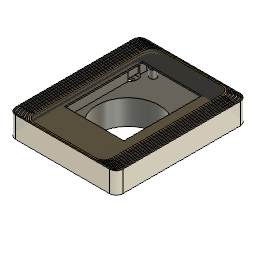
flush-mount-touch-display (Autodesk Fusion 360 design; units mm, degrees)
Autodesk Fusion 360 part; units mm, degrees
note: some values were not read from the file. Set by a fixed rule: which face or edge a step refers to.
(part 1 of 2)
sketch "Skizze2" plane through (0, 0, 0) normal (0, 0, 1) x (1, 0, 0)
  line L0 (0, 0) -> (50, 0)
  line L1 (50, 0) -> (50, 86)
  line L2 (50, 86) -> (0, 86)
  line L3 (0, 86) -> (0, 0)
  circle A0 centre (4.2, 5.1408) radius 1.25
  line L4 (25, 86) -> (25, 0) construction
  line L5 (0, 40) -> (50, 40) construction
  circle A1 centre (4.2, 5.1408) radius 2.5
  circle A2 centre (45.8, 5.1408) radius 1.25
  circle A3 centre (45.8, 5.1408) radius 2.5
  circle A4 centre (4.2, 82.6408) radius 1.25
  circle A5 centre (4.2, 82.6408) radius 2.5
  circle A6 centre (45.8, 82.6408) radius 2.5
  circle A7 centre (45.8, 82.6408) radius 1.25
  line L6 (43, 0) -> (7, 0)
  line L7 (7, 0) -> (7, 3.137)
  line L8 (7, 3.137) -> (43, 3.137)
  line L9 (43, 3.137) -> (43, 0)
  line L10 (43, 0) -> (7, 3.137) construction
  line L11 (7, 0) -> (43, 3.137) construction
  line L12 (50, 10) -> (0, 10) construction
  line L13 (0, 79.4) -> (50, 79.4) construction
  line L14 (0, 10) -> (0, 79.4) construction
  line L15 (0, 44.7) -> (50, 44.7) construction
  line L16 (2, -2) -> (48, -2)
  line L17 (52, 2) -> (52, 84)
  line L18 (48, 88) -> (2, 88)
  line L19 (-2, 84) -> (-2, 2)
  arc A8 (52, 84) -> (48, 88) centre (48, 84) ccw
  arc A9 (2, 88) -> (-2, 84) centre (2, 84) ccw
  arc A10 (-2, 2) -> (2, -2) centre (2, 2) ccw
  arc A11 (48, -2) -> (52, 2) centre (48, 2) ccw
  line L20 (-3.5, 84) -> (-3.5, 2)
  arc A12 (-3.5, 2) -> (2, -3.5) centre (2, 2) ccw
  line L21 (2, -3.5) -> (48, -3.5)
  arc A13 (48, -3.5) -> (53.5, 2) centre (48, 2) ccw
  line L22 (53.5, 2) -> (53.5, 84)
  arc A14 (53.5, 84) -> (48, 89.5) centre (48, 84) ccw
  line L23 (48, 89.5) -> (2, 89.5)
  arc A15 (2, 89.5) -> (-3.5, 84) centre (2, 84) ccw
  line L24 (7, 0) -> (7, -3.5)
  line L25 (43, 0) -> (43, -3.5)
  point P0 (25, 1.5685)
  dimension "d3" = 50
  dimension "d4" = 86
  dimension "d5" = 2.5
  dimension "d6" = 5
  dimension "d7" = 2.5
  dimension "d8" = 5
  dimension "d10" = 4
  dimension "d11" = 1.5
  dimension "d108" = 20.8
  dimension "d109" = 77.5
  dimension "d110" = 20.8
  constraint horizontal L0
  constraint vertical L1
  constraint horizontal L2
  constraint vertical L3
  constraint coincident L0.start L3.end
  constraint midpoint L2 L4.start
  constraint midpoint L0 L4.end
  constraint coincident L3 L5.start
  constraint coincident L1 L5.end
  constraint perpendicular L1 L5
  constraint concentric A0 A1
  constraint symmetric A0 L4 A2
  constraint symmetric L4 A1 A3
  constraint concentric A4 A5
  constraint symmetric L4 A4 A7
  constraint symmetric L4 A5 A6
  constraint horizontal L6
  constraint perpendicular L6 L7
  constraint parallel L6 L8
  constraint parallel L7 L9
  constraint coincident L10 P0
  constraint coincident L11 P0
  constraint coincident L0 L6.start
  constraint coincident L4 P0
  constraint coincident L1 L12.start
  constraint coincident L3 L12.end
  constraint perpendicular L3 L12
  constraint coincident L3 L13.start
  constraint coincident L1 L13.end
  constraint perpendicular L1 L13
  constraint midpoint L14 L15.start
  constraint coincident L1 L15.end
  constraint perpendicular L1 L15
  constraint tangent L17 A8
  constraint tangent L18 A8
  constraint tangent L18 A9
  constraint tangent L19 A9
  constraint equal A8 A9
  constraint tangent L16 A10
  constraint tangent L19 A10
  constraint equal A8 A10
  constraint tangent L16 A11
  constraint tangent L17 A11
  constraint equal A8 A11
  constraint coincident L21 L24.end
  constraint perpendicular L21 L24
  constraint coincident L21 L25.end
  constraint perpendicular L21 L25
  measures "d3" distance of L0.start L0.end
  measures "d4" distance of L0.start L2.end
  measures "d5" diameter of A0
  measures "d6" diameter of A1
  measures "d7" diameter of A4
  measures "d8" diameter of A5
  measures "d10" radius of A8
  measures "d108" distance of L4 A6.centre
  measures "d109" vertical distance of A2.centre A6.centre
  measures "d110" distance of L4 A2.centre
extrude "Extrusion1" add sketch "Skizze2" along normal blind 8.6 contours L16 L17 L18 L19 A8 A9 A10 A11 L20 A12 L21 A13 L22 A14 L23 A15 L24 L25 makes body 1
extrude "Extrusion2" add sketch "Skizze2" against normal blind 1.5 contours L0 L1 L2 L3 L7 L8 L9 | L0 L1 L2 L3 L16 L17 L18 L19 A8 A9 A10 A11 L24 L25 | L16 L17 L18 L19 A8 A9 A10 A11 L20 A12 L21 A13 L22 A14 L23 A15 L24 L25 | A0 | A1 | A2 | A3 | A4 | A5 | A6 | A7 bodies 1
extrude "Extrusion3" add sketch "Skizze2" along normal blind 4.2 contours A1 | A3 | A5 | A6 bodies 1
extrude "Extrusion4" add sketch "Skizze2" along normal blind 4.2 contours A0 | A2 | A4 | A7 bodies 1
sketch "Skizze3" plane through (0, 0, 0) normal (0, 0, 1) x (1, 0, 0)
  arc A0 (2, 89.5) -> (-3.5, 84) centre (2, 84) ccw
  line L0 (-3.5, 84) -> (-3.5, 2)
  arc A1 (-3.5, 2) -> (2, -3.5) centre (2, 2) ccw
  line L1 (2, -3.5) -> (48, -3.5)
  arc A2 (48, -3.5) -> (53.5, 2) centre (48, 2) ccw
  line L2 (53.5, 2) -> (53.5, 84)
  arc A3 (53.5, 84) -> (48, 89.5) centre (48, 84) ccw
  line L3 (48, 89.5) -> (2, 89.5)
  circle A4 centre (4.2, 82.6408) radius 2.5
  circle A5 centre (45.8, 82.6408) radius 2.5
  circle A6 centre (45.8, 5.1408) radius 2.5
  circle A7 centre (4.2, 5.1408) radius 2.5
  arc A8 (-3.55, 2) -> (2, -3.55) centre (2, 2) ccw
  line L4 (2, -3.55) -> (48, -3.55)
  arc A9 (48, -3.55) -> (53.55, 2) centre (48, 2) ccw
  line L5 (53.55, 2) -> (53.55, 84)
  arc A10 (53.55, 84) -> (48, 89.55) centre (48, 84) ccw
  line L6 (48, 89.55) -> (2, 89.55)
  arc A11 (2, 89.55) -> (-3.55, 84) centre (2, 84) ccw
  line L7 (-3.55, 84) -> (-3.55, 2)
  line L8 (48, 91.05) -> (2, 91.05)
  arc A12 (2, 91.05) -> (-5.05, 84) centre (2, 84) ccw
  line L9 (-5.05, 84) -> (-5.05, 2)
  arc A13 (-5.05, 2) -> (2, -5.05) centre (2, 2) ccw
  line L10 (2, -5.05) -> (48, -5.05)
  arc A14 (48, -5.05) -> (55.05, 2) centre (48, 2) ccw
  line L11 (55.05, 2) -> (55.05, 84)
  arc A15 (55.05, 84) -> (48, 91.05) centre (48, 84) ccw
  dimension "d26" = 0.05
  dimension "d27" = 1.55
extrude "Extrusion6" add sketch "Skizze3" against normal blind 1.8 separate body contours L8 A12 L9 A13 L10 A14 L11 A15 makes body 2
extrude "Extrusion7" add sketch "Skizze3" along normal blind 8.6 contours L8 A12 L9 A13 L10 A14 L11 A15 bodies 2
sketch "Skizze4" plane through (0, 0, 8.6) normal (0, 0, 1) x (-1, 0, 0)
  line L0 (3.55, -2) -> (3.55, -84)
  arc A0 (-2, -89.55) -> (3.55, -84) centre (-2, -84) ccw
  line L1 (-2, -89.55) -> (-48, -89.55)
  arc A1 (-53.55, -84) -> (-48, -89.55) centre (-48, -84) ccw
  line L2 (-53.55, -84) -> (-53.55, -2)
  arc A2 (-48, 3.55) -> (-53.55, -2) centre (-48, -2) ccw
  line L3 (-48, 3.55) -> (-2, 3.55)
  arc A3 (3.55, -2) -> (-2, 3.55) centre (-2, -2) ccw
  arc A4 (-55.05, -84) -> (-48, -91.05) centre (-48, -84) ccw
  line L4 (-48, -91.05) -> (-2, -91.05)
  arc A5 (-2, -91.05) -> (5.05, -84) centre (-2, -84) ccw
  line L5 (5.05, -84) -> (5.05, -2)
  arc A6 (5.05, -2) -> (-2, 5.05) centre (-2, -2) ccw
  line L6 (-2, 5.05) -> (-48, 5.05)
  arc A7 (-48, 5.05) -> (-55.05, -2) centre (-48, -2) ccw
  line L7 (-55.05, -2) -> (-55.05, -84)
  line L8 (5.05, -84) -> (5.05, -2)
  arc A8 (-2, -91.05) -> (5.05, -84) centre (-2, -84) ccw
  line L9 (-48, -91.05) -> (-2, -91.05)
  arc A9 (-55.05, -84) -> (-48, -91.05) centre (-48, -84) ccw
  line L10 (-55.05, -2) -> (-55.05, -84)
  arc A10 (-48, 5.05) -> (-55.05, -2) centre (-48, -2) ccw
  line L11 (-2, 5.05) -> (-48, 5.05)
  arc A11 (5.05, -2) -> (-2, 5.05) centre (-2, -2) ccw
  line L12 (0, -79.4) -> (-50, -79.4) construction
  line L13 (-50, -10) -> (0, -10) construction
  circle A12 centre (-4.2, -82.6408) radius 2.5
  circle A13 centre (-45.8, -82.6408) radius 2.5
  circle A14 centre (-45.8, -82.6408) radius 2.5
  circle A15 centre (-45.8, -5.1408) radius 2.5
  circle A16 centre (-45.8, -5.1408) radius 2.5
  circle A17 centre (-4.2, -5.1408) radius 2.5
  line L14 (0, -79.4) -> (0, -10) construction
  line L15 (-50, -79.4) -> (-50, -10) construction
  line L16 (0, -77.4) -> (-50, -77.4) construction
  line L17 (-50, -17.7) -> (0, -17.7) construction
  line L18 (-48, -79.4) -> (-48, -10) construction
  line L19 (-2, -79.4) -> (-2, -10) construction
  line L20 (-2, -77.4) -> (-48, -77.4)
  line L21 (-48, -77.4) -> (-48, -17.7)
  line L22 (-48, -17.7) -> (-2, -17.7)
  line L23 (-2, -17.7) -> (-2, -77.4)
  circle A18 centre (-45.8, -82.6408) radius 1.4
  circle A19 centre (-4.2, -82.6408) radius 1.4
  circle A20 centre (-45.8, -5.1408) radius 1.4
  circle A21 centre (-4.2, -5.1408) radius 1.4
  dimension "d32" = 2
  dimension "d33" = 7.7
  dimension "d34" = 2
  dimension "d35" = -2
  dimension "d44" = 2.8
  dimension "d45" = 2.8
  dimension "d46" = 2.8
  dimension "d47" = 2.8
  constraint coincident L12.start L14.start
  constraint coincident L13.end L14.end
  constraint coincident L12.end L15.start
  constraint coincident L13.start L15.end
  constraint horizontal L20
  constraint vertical L21
  constraint horizontal L22
  constraint vertical L23
  constraint coincident L18 L21.end
  constraint coincident L17 L21.end
  constraint coincident L19 L20.start
  constraint coincident L16 L20.start
  measures "d44" diameter of A18
  measures "d45" diameter of A19
  measures "d46" diameter of A20
  measures "d47" diameter of A21
extrude "Extrusion8" add sketch "Skizze4" along normal blind 1 contours L0 A0 L1 A1 L2 A2 L3 A3 | A4 L4 A5 L5 A6 L6 A7 L7 L8 A8 L9 A9 L10 A10 L11 A11 | A12 | A13 A14 | A15 A16 | A17 | A18 | A19 | A20 | A21 bodies 2
extrude "Extrusion9" add sketch "Skizze4" against normal blind 2.4 contours A12 | A13 A14 | A15 A16 | A17 | A18 | A19 | A20 | A21 bodies 2
sketch "Skizze5" plane through (0, 0, 9.6) normal (0, 0, 1) x (-1, 0, 0)
  line L0 (-48, -17.7) -> (-2, -17.7)
  line L1 (-2, -17.7) -> (-2, -77.4)
  line L2 (-2, -77.4) -> (-48, -77.4)
  line L3 (-48, -77.4) -> (-48, -17.7)
  arc A0 (5.05, -2) -> (-2, 5.05) centre (-2, -2) ccw
  line L4 (-2, 5.05) -> (-48, 5.05)
  arc A1 (-48, 5.05) -> (-55.05, -2) centre (-48, -2) ccw
  line L5 (-55.05, -2) -> (-55.05, -84)
  arc A2 (-55.05, -84) -> (-48, -91.05) centre (-48, -84) ccw
  line L6 (-48, -91.05) -> (-2, -91.05)
  arc A3 (-2, -91.05) -> (5.05, -84) centre (-2, -84) ccw
  line L7 (5.05, -84) -> (5.05, -2)
  line L8 (4.05, -84) -> (4.05, -2)
  arc A4 (4.05, -2) -> (-2, 4.05) centre (-2, -2) ccw
  line L9 (-2, 4.05) -> (-48, 4.05)
  arc A5 (-48, 4.05) -> (-54.05, -2) centre (-48, -2) ccw
  line L10 (-54.05, -2) -> (-54.05, -84)
  arc A6 (-54.05, -84) -> (-48, -90.05) centre (-48, -84) ccw
  line L11 (-48, -90.05) -> (-2, -90.05)
  arc A7 (-2, -90.05) -> (4.05, -84) centre (-2, -84) ccw
  line L12 (3.95, -84) -> (3.95, -2)
  arc A8 (3.95, -2) -> (-2, 3.95) centre (-2, -2) ccw
  line L13 (-2, 3.95) -> (-48, 3.95)
  arc A9 (-48, 3.95) -> (-53.95, -2) centre (-48, -2) ccw
  line L14 (-53.95, -2) -> (-53.95, -84)
  arc A10 (-53.95, -84) -> (-48, -89.95) centre (-48, -84) ccw
  line L15 (-48, -89.95) -> (-2, -89.95)
  arc A11 (-2, -89.95) -> (3.95, -84) centre (-2, -84) ccw
  dimension "d40" = -1
  dimension "d41" = -1.1
extrude "Extrusion10" cut sketch "Skizze5" against normal blind 0.1 contours L8 A4 L9 A5 L10 A6 L11 A7 bodies 2
sketch "Skizze6" plane through (0, 0, -1.5) normal (0, 0, -1) x (1, 0, 0)
  line L0 (7, -3.137) -> (7, 3.5)
  line L1 (7, 3.5) -> (2, 3.5)
  arc A0 (2, 3.5) -> (-3.5, -2) centre (2, -2) ccw
  line L2 (-3.5, -2) -> (-3.5, -84)
  arc A1 (-3.5, -84) -> (2, -89.5) centre (2, -84) ccw
  line L3 (2, -89.5) -> (48, -89.5)
  arc A2 (48, -89.5) -> (53.5, -84) centre (48, -84) ccw
  line L4 (53.5, -84) -> (53.5, -2)
  arc A3 (53.5, -2) -> (48, 3.5) centre (48, -2) ccw
  line L5 (48, 3.5) -> (43, 3.5)
  line L6 (43, 3.5) -> (43, -3.137)
  line L7 (43, -3.137) -> (7, -3.137)
  line L8 (2, 3.55) -> (48, 3.55)
  arc A4 (2, 3.55) -> (-3.55, -2) centre (2, -2) ccw
  arc A5 (53.55, -2) -> (48, 3.55) centre (48, -2) ccw
  line L9 (53.55, -2) -> (53.55, -84)
  arc A6 (48, -89.55) -> (53.55, -84) centre (48, -84) ccw
  line L10 (48, -89.55) -> (2, -89.55)
  arc A7 (-3.55, -84) -> (2, -89.55) centre (2, -84) ccw
  line L11 (-3.55, -84) -> (-3.55, -2)
  line L12 (25, 3.55) -> (25, -89.55) construction
  line L13 (-3.55, -43) -> (53.5, -43) construction
  line L14 (37, -79) -> (13, -79)
  line L15 (13, -79) -> (13, -7)
  line L16 (13, -7) -> (37, -7)
  line L17 (37, -7) -> (37, -79)
  line L18 (37, -79) -> (13, -7) construction
  line L19 (13, -79) -> (37, -7) construction
  circle A8 centre (28, -35) radius 3
  point P0 (25, -43)
  dimension "d49" = 24
  dimension "d121" = 6
  constraint midpoint L8 L12.start
  constraint midpoint L10 L12.end
  constraint midpoint L11 L13.start
  constraint midpoint L4 L13.end
  constraint horizontal L14
  constraint perpendicular L14 L15
  constraint parallel L14 L16
  constraint parallel L15 L17
  constraint coincident L18 P0
  constraint coincident L19 P0
  constraint midpoint L12 P0
  measures "d49" distance of L15.end L16.end
  measures "d121" diameter of A8
extrude "Extrusion11" add sketch "Skizze6" along normal blind 22 contours L14 L15 L16 L17 | A8 bodies 1
sketch "Skizze7" plane through (0, 79, 0) normal (0, 1, 0) x (-1, 0, 0)
  line L0 (-13, -1.5) -> (-37, -1.5)
  line L1 (-37, -1.5) -> (-37, -23.5)
  line L2 (-37, -23.5) -> (-13, -23.5)
  line L3 (-13, -23.5) -> (-13, -1.5)
  line L4 (-25, -23.5) -> (-25, -1.5) construction
  circle A0 centre (-25, -17) radius 12
  dimension "d52" = 24
  constraint midpoint L2 L4.start
  constraint midpoint L0 L4.end
  constraint coincident L4 A0.centre
  measures "d52" diameter of A0
extrude "Extrusion12" cut 1 faces at (21, 31, -23.5) along direction (0, 0, 1) blind 7 on bodies 1 bodies 1
fillet "Abrundung1" radius 12 1 edges at (25, 79, -16.5) on bodies 1
fillet "Abrundung2" radius 12 1 edges at (25, 7, -16.5) on bodies 1
extrude "Extrusion13" cut sketch "Skizze7" against normal blind 79 contours L2 A0 | L2 A0 bodies 1
sketch "Skizze16" plane through (0, 0, 0) normal (0, 0, 1) x (1, 0, 0)
  line L0 (37, 61) -> (13, 61)
  line L1 (13, 61) -> (13, 65)
  line L2 (13, 65) -> (37, 65)
  line L3 (37, 65) -> (37, 61)
  line L4 (37, 61) -> (13, 65) construction
  line L5 (13, 61) -> (37, 65) construction
  line L6 (37, 21) -> (13, 21)
  line L7 (13, 21) -> (13, 25)
  line L8 (13, 25) -> (37, 25)
  line L9 (37, 25) -> (37, 21)
  line L10 (37, 21) -> (13, 25) construction
  line L11 (13, 21) -> (37, 25) construction
  circle A0 centre (28, 35) radius 3
  line L12 (28, 38) -> (34, 38)
  line L13 (34, 38) -> (34, 32)
  line L14 (34, 32) -> (28, 32)
  line L15 (28, 32) -> (28, 38)
  line L16 (28, 38) -> (16, 38)
  line L17 (16, 38) -> (16, 32)
  line L18 (16, 32) -> (28, 32)
  line L19 (28, 32) -> (28, 38)
  point P0 (25, 63)
  point P1 (25, 23)
  constraint horizontal L0
  constraint perpendicular L0 L1
  constraint parallel L0 L2
  constraint parallel L1 L3
  constraint coincident L4 P0
  constraint coincident L5 P0
  constraint horizontal L6
  constraint perpendicular L6 L7
  constraint parallel L6 L8
  constraint parallel L7 L9
  constraint coincident L10 P1
  constraint coincident L11 P1
  constraint horizontal L12
  constraint vertical L13
  constraint horizontal L14
  constraint vertical L15
  constraint coincident A0 L12.start
  constraint horizontal L16
  constraint vertical L17
  constraint horizontal L18
  constraint vertical L19
extrude "Extrusion25" add 1 faces at (-3, 56.6667, 8.6) along direction (0, 0, 1) blind 0.9 on bodies 1 bodies 1
move_body "Verschieben1" bodies 2 to x (1, 0, 0) y (0, 1, 0) z (0, 0, 1) at (0, 0, 0.9)
extrude "Extrusion26" add 1 faces at (54.55, 29.3333, -0.9) along direction (0, 0, -1) blind 0.9 on bodies 2 bodies 2
extrude "Extrusion27" add sketch "Skizze2" along normal blind 8 contours A0 | A2 | A4 | A7 bodies 1
extrude "Extrusion28" add sketch "Skizze4" along normal blind 1 contours A12 | A13 A14 | A15 A16 | A17 bodies 2
extrude "Extrusion29" add sketch "Skizze4" against normal blind 2.8 contours A12 | A13 A14 | A15 A16 | A17 bodies 2
sketch "Skizze17" plane through (0, 0, 0) normal (0, 0, 1) x (1, 0, 0)
  line L0 (17, 32, -33) -> (33, 32, -33)
  line L1 (33, 32, -33) -> (33, 38, -33)
  line L2 (33, 38, -33) -> (17, 38, -33)
  line L3 (17, 38, -33) -> (17, 32, -33)
extrude "Extrusion34" cut 4 faces at (3.9935, 4.8544, 7.1) (3.9667, 82.2367, 7.1) (45.5667, 83.045, 7.1) (46.4103, 4.7622, 7.1) along direction (0, 0, 1) blind 1.5 on bodies 2 bodies 2
copy_body "Körper->Berechn1" bodies 1 removing the originals makes body 3 in component "Inner Body"
copy_body "Körper->Berechn2" bodies 2 removing the originals makes body 4 in component "Outer Body"
sketch "Skizze18" plane through (0, 0, 0) normal (0, 1, 0) x (1, 0, 0)
sketch "Skizze19" plane through (-5.05, 0, 0) normal (-1, 0, 0) x (0, -1, 0)
  line L0 (-84, 10.5) -> (-84, -1.8)
  line L1 (-84, -1.8) -> (-2, -1.8)
  line L2 (-2, -1.8) -> (-2, 10.5)
  line L3 (-2, 10.5) -> (-84, 10.5)
delete_face "Fläche löschen1" 1 faces at (37, 35, -6.5) on bodies 3 in component "Inner Body"
sketch "Skizze20" plane through (0, 0, 0) normal (0, 0, 1) x (-1, 0, 0)
  circle A0 centre (-4.2, -82.6408) radius 2.5
  circle A1 centre (-45.8, -82.6408) radius 2.5
  line L0 (-2, 2) -> (-7, 2)
  line L1 (-7, 2) -> (-7, -3.137)
  line L2 (-7, -3.137) -> (-43, -3.137)
  line L3 (-43, -3.137) -> (-43, 2)
  line L4 (-43, 2) -> (-48, 2)
  arc A2 (-48, 2) -> (-52, -2) centre (-48, -2) ccw
  line L5 (-52, -2) -> (-52, -84)
  arc A3 (-52, -84) -> (-48, -88) centre (-48, -84) ccw
  line L6 (-48, -88) -> (-2, -88)
  arc A4 (-2, -88) -> (2, -84) centre (-2, -84) ccw
  line L7 (2, -84) -> (2, -2)
  arc A5 (2, -2) -> (-2, 2) centre (-2, -2) ccw
  circle A6 centre (-4.2, -5.1408) radius 2.5
  circle A7 centre (-45.8, -5.1408) radius 2.5
  circle A8 centre (-25, -43.4454) radius 6
  line L8 (-4.2, -82.6408) -> (-12.2, -82.6408) construction
  line L9 (-12.2, -82.6408) -> (-12.2, -74.6408) construction
  circle A9 centre (-12.2, -74.6408) radius 2.1
  line L10 (-25, -88) -> (-25, -5.1408) construction
  line L11 (-4.2, -5.1408) -> (-12.2, -5.1408) construction
  line L12 (-12.2, -5.1408) -> (-12.2, -13.1408) construction
  circle A10 centre (-12.2, -13.1408) radius 2.1
  circle A11 centre (-37.8, -13.1408) radius 2.1
  circle A12 centre (-37.8, -74.6408) radius 2.1
  dimension "d152" = 12
  dimension "d155" = 8
  dimension "d156" = 8
  dimension "d157" = 4.2
  dimension "d158" = 8
  dimension "d159" = 8
  dimension "d160" = 4.2
  constraint coincident A0.centre L8.start
  constraint perpendicular L8 L9
  constraint coincident L9.end A9.centre
  constraint midpoint L6 L10.start
  constraint perpendicular L2 L10
  constraint coincident A6.centre L11.start
  constraint perpendicular L7 L11
  constraint perpendicular L11 L12
  constraint coincident L12.end A10.centre
  constraint symmetric A9 L10 A12
  constraint symmetric L10 A10 A11
  measures "d152" diameter of A8
  measures "d155" distance of A0.centre L8.end
  measures "d156" distance of L8.end L9.end
  measures "d157" diameter of A9
  measures "d158" distance of A6.centre L11.end
  measures "d159" distance of L11.end L12.end
  measures "d160" diameter of A10
extrude "Extrusion2'" cut sketch "Skizze20" against normal blind 5 contours A8 | A9 | A10 | A11 | A12 bodies 3 in component "Inner Body"
sketch "Skizze21" plane through (0, 0, 0) normal (0, 0, 1) x (-1, 0, 0)
  circle A0 centre (-25, -43.4454) radius 6
  circle A1 centre (-37.8, -74.6408) radius 2.1
  circle A2 centre (-37.8, -13.1408) radius 2.1
  circle A3 centre (-12.2, -74.6408) radius 2.1
  circle A4 centre (-12.2, -13.1408) radius 2.1
  circle A5 centre (-4.2, -82.6408) radius 2.5
  circle A6 centre (-45.8, -82.6408) radius 2.5
  line L0 (-2, 2) -> (-7, 2)
  line L1 (-7, 2) -> (-7, -3.137)
  line L2 (-7, -3.137) -> (-43, -3.137)
  line L3 (-43, -3.137) -> (-43, 2)
  line L4 (-43, 2) -> (-48, 2)
  arc A7 (-48, 2) -> (-52, -2) centre (-48, -2) ccw
  line L5 (-52, -2) -> (-52, -84)
  arc A8 (-52, -84) -> (-48, -88) centre (-48, -84) ccw
  line L6 (-48, -88) -> (-2, -88)
  arc A9 (-2, -88) -> (2, -84) centre (-2, -84) ccw
  line L7 (2, -84) -> (2, -2)
  arc A10 (2, -2) -> (-2, 2) centre (-2, -2) ccw
  circle A11 centre (-4.2, -5.1408) radius 2.5
  circle A12 centre (-45.8, -5.1408) radius 2.5
  line L8 (-25, -88) -> (-25, 3) construction
  line L9 (-52, -43) -> (2, -43) construction
  line L10 (5.45, -7.55) -> (-55.45, -7.55)
  line L11 (-60.45, -12.55) -> (-60.45, -73.45)
  line L12 (-55.45, -78.45) -> (5.45, -78.45)
  line L13 (10.45, -73.45) -> (10.45, -12.55)
  line L14 (10.45, -7.55) -> (-60.45, -78.45) construction
  line L15 (-60.45, -7.55) -> (10.45, -78.45) construction
  arc A13 (-60.45, -73.45) -> (-55.45, -78.45) centre (-55.45, -73.45) ccw
  arc A14 (5.45, -78.45) -> (10.45, -73.45) centre (5.45, -73.45) ccw
  arc A15 (10.45, -12.55) -> (5.45, -7.55) centre (5.45, -12.55) ccw
  arc A16 (-55.45, -7.55) -> (-60.45, -12.55) centre (-55.45, -12.55) ccw
  line L16 (3.55, -84) -> (3.55, -2)
  arc A17 (3.55, -2) -> (-2, 3.55) centre (-2, -2) ccw
  line L17 (-2, 3.55) -> (-48, 3.55)
  arc A18 (-48, 3.55) -> (-53.55, -2) centre (-48, -2) ccw
  line L18 (-53.55, -2) -> (-53.55, -84)
  arc A19 (-53.55, -84) -> (-48, -89.55) centre (-48, -84) ccw
  line L19 (-48, -89.55) -> (-2, -89.55)
  arc A20 (-2, -89.55) -> (3.55, -84) centre (-2, -84) ccw
  arc A21 (-55.05, -84) -> (-48, -91.05) centre (-48, -84) ccw
  line L20 (-55.05, -84) -> (-55.05, -2)
  arc A22 (-48, 5.05) -> (-55.05, -2) centre (-48, -2) ccw
  line L21 (-48, 5.05) -> (-2, 5.05)
  arc A23 (5.05, -2) -> (-2, 5.05) centre (-2, -2) ccw
  line L22 (5.05, -2) -> (5.05, -84)
  arc A24 (-2, -91.05) -> (5.05, -84) centre (-2, -84) ccw
  line L23 (-2, -91.05) -> (-48, -91.05)
  line L24 (-65.25, -83.25) -> (15.25, -83.25)
  line L25 (15.25, -83.25) -> (15.25, -2.75)
  line L26 (15.25, -2.75) -> (-65.25, -2.75)
  line L27 (-65.25, -2.75) -> (-65.25, -83.25)
  line L28 (-65.25, -83.25) -> (15.25, -2.75) construction
  line L29 (15.25, -83.25) -> (-65.25, -2.75) construction
  line L30 (-60.25, -92.0661) -> (10.25, -92.0661)
  line L31 (15.25, -87.0661) -> (15.25, 1.0661)
  line L32 (10.25, 6.0661) -> (-60.25, 6.0661)
  line L33 (-65.25, 1.0661) -> (-65.25, -87.0661)
  line L34 (-65.25, -92.0661) -> (15.25, 6.0661) construction
  line L35 (15.25, -92.0661) -> (-65.25, 6.0661) construction
  arc A25 (10.25, -92.0661) -> (15.25, -87.0661) centre (10.25, -87.0661) ccw
  arc A26 (-65.25, -87.0661) -> (-60.25, -92.0661) centre (-60.25, -87.0661) ccw
  arc A27 (-60.25, 6.0661) -> (-65.25, 1.0661) centre (-60.25, 1.0661) ccw
  arc A28 (15.25, 1.0661) -> (10.25, 6.0661) centre (10.25, 1.0661) ccw
  line L36 (-55.23, -84) -> (-55.23, -2)
  arc A29 (-48, 5.23) -> (-55.23, -2) centre (-48, -2) ccw
  line L37 (-48, 5.23) -> (-2, 5.23)
  arc A30 (5.23, -2) -> (-2, 5.23) centre (-2, -2) ccw
  line L38 (5.23, -2) -> (5.23, -84)
  arc A31 (-2, -91.23) -> (5.23, -84) centre (-2, -84) ccw
  line L39 (-2, -91.23) -> (-48, -91.23)
  arc A32 (-55.23, -84) -> (-48, -91.23) centre (-48, -84) ccw
  circle A33 centre (-25, -43) radius 26.75
  point P0 (-25, -43.8908)
  point P1 (-25, -43.8908)
  point P2 (-25, -43)
  point P3 (-25, -43)
  point P4 (-25, -43)
  dimension "d167" = 70.9
  dimension "d168" = 70.9
  dimension "d169" = 5
  dimension "d170" = 80.5
  dimension "d171" = 80.5
  dimension "d172" = 5
  dimension "d173" = 0.18
  dimension "d180" = 53.5
  constraint coincident P1 P0
  constraint midpoint L6 L8.start
  constraint perpendicular L2 L8
  constraint midpoint L5 L9.start
  constraint midpoint L7 L9.end
  constraint horizontal L10
  constraint perpendicular L10 L11
  constraint parallel L10 L12
  constraint parallel L11 L13
  constraint coincident L14 P4
  constraint coincident L15 P4
  constraint midpoint L9 P4
  constraint coincident L14.end L11
  constraint coincident L14.end L12
  constraint tangent L11 A13
  constraint tangent L12 A13
  constraint coincident L15.end L12
  constraint coincident L15.end L13
  constraint tangent L12 A14
  constraint tangent L13 A14
  constraint equal A13 A14
  constraint coincident L14.start L10
  constraint coincident L14.start L13
  constraint tangent L10 A15
  constraint tangent L13 A15
  constraint equal A13 A15
  constraint coincident L15.start L10
  constraint coincident L15.start L11
  constraint tangent L10 A16
  constraint tangent L11 A16
  constraint equal A13 A16
  constraint horizontal L24
  constraint perpendicular L24 L25
  constraint parallel L24 L26
  constraint parallel L25 L27
  constraint coincident L28 P4
  constraint coincident L29 P4
  constraint coincident P4 P3
  constraint horizontal L30
  constraint perpendicular L30 L31
  constraint parallel L30 L32
  constraint parallel L31 L33
  constraint coincident L34 P4
  constraint coincident L35 P4
  constraint coincident L35.start L30
  constraint coincident L35.start L31
  constraint tangent L30 A25
  constraint tangent L31 A25
  constraint coincident L34.start L33
  constraint coincident L34.start L30
  constraint tangent L33 A26
  constraint tangent L30 A26
  constraint equal A25 A26
  constraint coincident L35.end L33
  constraint coincident L35.end L32
  constraint tangent L33 A27
  constraint tangent L32 A27
  constraint equal A25 A27
  constraint coincident L34.end L32
  constraint coincident L34.end L31
  constraint tangent L32 A28
  constraint tangent L31 A28
  constraint equal A25 A28
  measures "d167" distance of L14.end L15.end
  measures "d168" distance of L15.start L14.end
  measures "d169" radius of A13
  measures "d170" distance of L25.end L26.end
  measures "d171" distance of L24.end L25.end
  measures "d172" radius of A25
  measures "d180" diameter of A33
extrude "Extrusion37" add sketch "Skizze21" against normal blind 2.5 separate body contours A0 | A1 | A2 | A3 | A4 | A5 L24 | A5 A6 L5 L7 L12 L24 | A5 L24 | A5 A6 L5 A8 L6 A9 L7 L24 | A6 L24 | A6 L24 | L5 A8 L6 A9 L7 L16 L18 A19 L19 A20 L24 | L7 L12 L16 L24 | L5 L7 A11 A12 L10 L12 | L7 L10 L12 L16 | L16 L18 A19 L19 A20 A21 L20 L22 A24 L23 L24 | L12 L16 L22 L24 | L5 L12 L18 L24 | L7 A11 L10 L26 | L7 L10 L16 L26 | L5 L10 L12 L18 | L10 L12 L16 L22 | A21 L20 L22 A24 L23 L24 L36 L38 A31 L39 A32 | L12 L22 L24 L38 | L12 L18 L20 L24 | L0 L1 L7 A10 A11 L26 | L0 L1 L3 L4 A7 L5 L7 A10 L16 A17 L17 A18 L18 L26 | L10 L16 L22 L26 | A11 L10 L26 | A11 L10 | L5 L10 L18 L26 | L5 A12 L10 L26 | L10 L12 L18 L20 | L10 L12 L22 L38 | L10 L12 L13 A14 A15 L24 L25 L26 L31 L38 | L24 L30 L31 L33 A25 A26 L36 L38 A31 L39 A32 | L12 L20 L24 L36 | L16 A17 L17 A18 L18 L20 A22 L21 A23 L22 L26 | A11 L26 | L10 L22 L26 L38 | L1 L2 L3 A11 A12 L10 L26 | L3 L4 A7 L5 A12 L26 | A12 L10 | A12 L10 L26 | L10 L18 L20 L26 | L10 L12 L20 L36 | L10 L12 L13 A14 A15 L38 | L10 L11 L12 A13 A16 L24 L26 L27 L33 L36 | L20 A22 L21 A23 L22 L26 L36 A29 L37 A30 L38 | A12 L26 | L10 L20 L26 L36 | L10 L11 L12 A13 A16 L36 | L26 L31 L32 L33 A27 A28 L36 A29 L37 A30 L38 | L1 L2 L3 L26 | A33 makes body 5
extrude "Extrusion38" cut sketch "Skizze21" against normal blind 1.8 contours L16 L18 A19 L19 A20 A21 L20 L22 A24 L23 L24 | L12 L16 L22 L24 | L10 L12 L16 L22 | L12 L18 L20 L24 | L10 L16 L22 L26 | L10 L12 L18 L20 | L16 A17 L17 A18 L18 L20 A22 L21 A23 L22 L26 | L10 L18 L20 L26 bodies 5
extrude "Extrusion39" cut sketch "Skizze21" against normal blind 18 contours A0 | A33 bodies 5
extrude "Extrusion3'" cut sketch "Skizze21" against normal blind 18 contours A0 | A33 bodies 3 in component "Inner Body"
sketch "Skizze22" plane through (0, 0, -2.5) normal (0, 0, -1) x (1, 0, 0)
  circle A0 centre (25, -43) radius 26.75
  line L0 (60.25, 6.0661) -> (-10.25, 6.0661)
  arc A1 (-10.25, 6.0661) -> (-15.25, 1.0661) centre (-10.25, 1.0661) ccw
  line L1 (-15.25, 1.0661) -> (-15.25, -87.0661)
  arc A2 (-15.25, -87.0661) -> (-10.25, -92.0661) centre (-10.25, -87.0661) ccw
  line L2 (-10.25, -92.0661) -> (60.25, -92.0661)
  arc A3 (60.25, -92.0661) -> (65.25, -87.0661) centre (60.25, -87.0661) ccw
  line L3 (65.25, -87.0661) -> (65.25, 1.0661)
  arc A4 (65.25, 1.0661) -> (60.25, 6.0661) centre (60.25, 1.0661) ccw
  line L4 (60.45, -12.55) -> (60.45, -73.45)
  arc A5 (55.45, -78.45) -> (60.45, -73.45) centre (55.45, -73.45) ccw
  line L5 (55.45, -78.45) -> (-5.45, -78.45)
  arc A6 (-10.45, -73.45) -> (-5.45, -78.45) centre (-5.45, -73.45) ccw
  line L6 (-10.45, -73.45) -> (-10.45, -12.55)
  arc A7 (-5.45, -7.55) -> (-10.45, -12.55) centre (-5.45, -12.55) ccw
  line L7 (-5.45, -7.55) -> (55.45, -7.55)
  arc A8 (60.45, -12.55) -> (55.45, -7.55) centre (55.45, -12.55) ccw
  circle A9 centre (25, -43) radius 26.75
  ellipse E0 centre (55.45, -73.45) end of major axis (53, -76) minor radius 1.9
  line L8 (57.9, -70.9) -> (53, -76) construction
  line L9 (54.0799, -72.1336) -> (56.8201, -74.7664) construction
  ellipse E1 centre (55.45, -12.55) end of major axis (58, -15) minor radius 1.9
  ellipse E2 centre (-5.45, -12.55) end of major axis (-3, -10) minor radius 1.9
  ellipse E3 centre (-5.45, -73.45) end of major axis (-8, -71) minor radius 1.9
  dimension "d185" = 3.8
  dimension "d187" = 360
  constraint coincident E0 L8.start
  constraint coincident E0 L8.end
  constraint coincident E0 L9.start
  constraint coincident E0 L9.end
  constraint concentric A5 E0
extrude "Extrusion40" add sketch "Skizze22" along normal blind 3 contours L0 A1 L1 A2 L2 A3 L3 A4 | L4 A5 L5 A6 L6 A7 L7 A8 bodies 5
sketch "Skizze23" plane through (0, 0, 0) normal (0, 0, 1) x (-1, 0, 0)
  arc A0 (-60.25, 6.0661) -> (-65.25, 1.0661) centre (-60.25, 1.0661) ccw
  line L0 (-65.25, 1.0661) -> (-65.25, -87.0661)
  arc A1 (-65.25, -87.0661) -> (-60.25, -92.0661) centre (-60.25, -87.0661) ccw
  line L1 (-60.25, -92.0661) -> (10.25, -92.0661)
  arc A2 (10.25, -92.0661) -> (15.25, -87.0661) centre (10.25, -87.0661) ccw
  line L2 (15.25, -87.0661) -> (15.25, 1.0661)
  arc A3 (15.25, 1.0661) -> (10.25, 6.0661) centre (10.25, 1.0661) ccw
  line L3 (10.25, 6.0661) -> (-60.25, 6.0661)
  line L4 (-48, 5.05) -> (-2, 5.05)
  arc A4 (5.05, -2) -> (-2, 5.05) centre (-2, -2) ccw
  line L5 (5.05, -2) -> (5.05, -84)
  arc A5 (-2, -91.05) -> (5.05, -84) centre (-2, -84) ccw
  line L6 (-2, -91.05) -> (-48, -91.05)
  arc A6 (-55.05, -84) -> (-48, -91.05) centre (-48, -84) ccw
  line L7 (-55.05, -84) -> (-55.05, -2)
  arc A7 (-48, 5.05) -> (-55.05, -2) centre (-48, -2) ccw
  ellipse E0 centre (5.45, -12.55) end of major axis (3, -10) minor radius 1.9
  ellipse E1 centre (-55.45, -12.55) end of major axis (-58, -15) minor radius 1.9
  ellipse E2 centre (-55.45, -73.45) end of major axis (-53, -76) minor radius 1.9
  ellipse E3 centre (5.45, -73.45) end of major axis (8, -71) minor radius 1.9
  ellipse E4 centre (5.45, -73.45) end of major axis (10.1633, -68.9215) minor radius 4.9
  ellipse E5 centre (-55.45, -73.45) end of major axis (-50.9215, -78.1633) minor radius 4.9
  ellipse E6 centre (-55.45, -12.55) end of major axis (-60.1633, -17.0785) minor radius 4.9
  ellipse E7 centre (5.45, -12.55) end of major axis (0.9215, -7.8367) minor radius 4.9
extrude "Extrusion41" cut sketch "Skizze23" against normal blind 4 contours L7 E1 E6 | L7 E1 E6 | L5 E0 E7 | L5 E0 E7 | L7 E1 | L7 E1 | L5 E0 | L5 E0 | L7 E2 E5 | L7 E2 E5 | L5 E3 E4 | L5 E3 E4 | L7 E2 | L7 E2 | L5 E3 | L5 E3 bodies 5
extrude "Extrusion4'" cut sketch "Skizze23" along normal blind 11 and the other way blind 4 contours L7 E1 E6 | L7 E1 E6 | L5 E0 E7 | L5 E0 E7 | L7 E1 | L7 E1 | L5 E0 | L5 E0 | L7 E2 E5 | L7 E2 E5 | L5 E3 E4 | L5 E3 E4 | L7 E2 | L7 E2 | L5 E3 | L5 E3 bodies 3 in component "Inner Body"
sketch "Skizze24" plane through (0, 0, -5.5) normal (0, 0, -1) x (1, 0, 0)
  ellipse E0 centre (-5.45, -12.55) end of major axis (-3, -10) minor radius 1.9
  ellipse E1 centre (-5.45, -73.45) end of major axis (-8, -71) minor radius 1.9
  circle A0 centre (25, -43) radius 26.75
  ellipse E2 centre (55.45, -12.55) end of major axis (58, -15) minor radius 1.9
  ellipse E3 centre (55.45, -73.45) end of major axis (53, -76) minor radius 1.9
  arc A1 (65.25, 1.0661) -> (60.25, 6.0661) centre (60.25, 1.0661) ccw
  line L0 (60.25, 6.0661) -> (-10.25, 6.0661)
  arc A2 (-10.25, 6.0661) -> (-15.25, 1.0661) centre (-10.25, 1.0661) ccw
  line L1 (-15.25, 1.0661) -> (-15.25, -87.0661)
  arc A3 (-15.25, -87.0661) -> (-10.25, -92.0661) centre (-10.25, -87.0661) ccw
  line L2 (-10.25, -92.0661) -> (60.25, -92.0661)
  arc A4 (60.25, -92.0661) -> (65.25, -87.0661) centre (60.25, -87.0661) ccw
  line L3 (65.25, -87.0661) -> (65.25, 1.0661)
  circle A5 centre (25, -43) radius 26.75
  circle A6 centre (25, -43) radius 28.75
  dimension "d196" = 2
extrude "Extrusion42" add sketch "Skizze24" along normal blind 30 contours A6 bodies 5
sketch "Skizze25" plane through (0, 0, -35.5) normal (0, 0, -1) x (1, 0, 0)
  circle A0 centre (25, -43) radius 26.75
  circle A1 centre (25, -43) radius 28.75
  circle A2 centre (25, -43) radius 28.75
  circle A3 centre (25, -43) radius 15
  dimension "d201" = 30
  constraint concentric A2 A3
  measures "d201" diameter of A3
extrude "Extrusion43" add sketch "Skizze25" against normal blind 2 contours A0 | A1 A2 | A3 bodies 5
extrude "Extrusion44" cut sketch "Skizze25" against normal blind 11 contours A3 bodies 5
extrude "Extrusion45" cut 1 faces at (59.4089, 3.0609, 0) along direction (0, 0, -1) blind 1.9 on bodies 5 bodies 5
extrude "Extrusion46" add 1 faces at (59.4089, 3.0609, -1.9) along direction (0, 0, 1) blind 0.1 on bodies 5 bodies 5
sketch "Skizze26" plane through (0, 0, -1.8) normal (0, 0, 1) x (-1, 0, 0)
  arc A0 (15.25, 1.0661) -> (10.25, 6.0661) centre (10.25, 1.0661) ccw
  line L0 (10.25, 6.0661) -> (-60.25, 6.0661)
  arc A1 (-60.25, 6.0661) -> (-65.25, 1.0661) centre (-60.25, 1.0661) ccw
  line L1 (-65.25, 1.0661) -> (-65.25, -87.0661)
  arc A2 (-65.25, -87.0661) -> (-60.25, -92.0661) centre (-60.25, -87.0661) ccw
  line L2 (-60.25, -92.0661) -> (10.25, -92.0661)
  arc A3 (10.25, -92.0661) -> (15.25, -87.0661) centre (10.25, -87.0661) ccw
  line L3 (15.25, -87.0661) -> (15.25, 1.0661)
  ellipse E0 centre (-55.45, -12.55) end of major axis (-60.1633, -17.0785) minor radius 4.9 (-53.55, -6.8131) -> (-53.55, -17.234) ccw
  line L4 (-53.55, -6.8131) -> (-53.55, -2)
  arc A4 (-48, 3.55) -> (-53.55, -2) centre (-48, -2) ccw
  line L5 (-48, 3.55) -> (-2, 3.55)
  arc A5 (3.55, -2) -> (-2, 3.55) centre (-2, -2) ccw
  line L6 (3.55, -2) -> (3.55, -6.7496)
  ellipse E1 centre (5.45, -12.55) end of major axis (0.9215, -7.8367) minor radius 4.9 (3.55, -17.2737) -> (3.55, -6.7496) ccw
  line L7 (3.55, -17.2737) -> (3.55, -68.766)
  ellipse E2 centre (5.45, -73.45) end of major axis (10.1633, -68.9215) minor radius 4.9 (3.55, -79.1869) -> (3.55, -68.766) ccw
  line L8 (3.55, -79.1869) -> (3.55, -84)
  arc A6 (-2, -89.55) -> (3.55, -84) centre (-2, -84) ccw
  line L9 (-2, -89.55) -> (-48, -89.55)
  arc A7 (-53.55, -84) -> (-48, -89.55) centre (-48, -84) ccw
  line L10 (-53.55, -84) -> (-53.55, -79.2504)
  ellipse E3 centre (-55.45, -73.45) end of major axis (-50.9215, -78.1633) minor radius 4.9 (-53.55, -68.7263) -> (-53.55, -79.2504) ccw
  line L11 (-53.55, -68.7263) -> (-53.55, -17.234)
sketch "Skizze27" plane through (0, 0, 10.5) normal (0, 0, 1) x (-1, 0, 0)
  line L0 (-48, -89.95) -> (-2, -89.95)
  arc A0 (-2, -89.95) -> (3.95, -84) centre (-2, -84) ccw
  line L1 (3.95, -84) -> (3.95, -2)
  arc A1 (3.95, -2) -> (-2, 3.95) centre (-2, -2) ccw
  line L2 (-2, 3.95) -> (-48, 3.95)
  arc A2 (-48, 3.95) -> (-53.95, -2) centre (-48, -2) ccw
  line L3 (-53.95, -2) -> (-53.95, -84)
  arc A3 (-53.95, -84) -> (-48, -89.95) centre (-48, -84) ccw
  line L4 (-48, -17.7) -> (-2, -17.7)
  line L5 (-2, -17.7) -> (-2, -77.4)
  line L6 (-2, -77.4) -> (-48, -77.4)
  line L7 (-48, -77.4) -> (-48, -17.7)
  line L8 (10.25, 6.0661) -> (-60.25, 6.0661)
  arc A4 (-60.25, 6.0661) -> (-65.25, 1.0661) centre (-60.25, 1.0661) ccw
  line L9 (-65.25, 1.0661) -> (-65.25, -87.0661)
  arc A5 (-65.25, -87.0661) -> (-60.25, -92.0661) centre (-60.25, -87.0661) ccw
  line L10 (-60.25, -92.0661) -> (10.25, -92.0661)
  arc A6 (10.25, -92.0661) -> (15.25, -87.0661) centre (10.25, -87.0661) ccw
  line L11 (15.25, -87.0661) -> (15.25, 1.0661)
  arc A7 (15.25, 1.0661) -> (10.25, 6.0661) centre (10.25, 1.0661) ccw
  arc A8 (5.05, -2) -> (-2, 5.05) centre (-2, -2) ccw
  line L12 (-2, 5.05) -> (-48, 5.05)
  arc A9 (-48, 5.05) -> (-55.05, -2) centre (-48, -2) ccw
  line L13 (-55.05, -2) -> (-55.05, -84)
  arc A10 (-55.05, -84) -> (-48, -91.05) centre (-48, -84) ccw
  line L14 (-48, -91.05) -> (-2, -91.05)
  arc A11 (-2, -91.05) -> (5.05, -84) centre (-2, -84) ccw
  line L15 (5.05, -84) -> (5.05, -2)
  line L16 (4.05, -2) -> (4.05, -84)
  arc A12 (-2, -90.05) -> (4.05, -84) centre (-2, -84) ccw
  line L17 (-2, -90.05) -> (-48, -90.05)
  arc A13 (-54.05, -84) -> (-48, -90.05) centre (-48, -84) ccw
  line L18 (-54.05, -84) -> (-54.05, -2)
  arc A14 (-48, 4.05) -> (-54.05, -2) centre (-48, -2) ccw
  line L19 (-48, 4.05) -> (-2, 4.05)
  arc A15 (4.05, -2) -> (-2, 4.05) centre (-2, -2) ccw
extrude "Extrusion1'" add sketch "Skizze27" against normal blind 12.3 contours L8 A4 L9 A5 L10 A6 L11 A7 bodies 4 in component "Outer Body"
extrude "Extrusion2''" add sketch "Skizze27" along normal blind 0.5 contours A8 L12 A9 L13 A10 L14 A11 L15 bodies 4 in component "Outer Body"
combine "Kombinieren1" operation add target body 5 tool bodies 3
extrude "Extrusion3''" cut 1 faces at (54.7167, 29.3333, 11) along direction (0, 0, -1) blind 0.4 on bodies 4 bodies 4 in component "Outer Body"
extrude "Extrusion47" cut 1 faces at (32.6667, 89.5167, 0) along direction (0, 0, -1) blind 1.8 on bodies 5 bodies 5
extrude "Extrusion48" cut 1 faces at (53.5292, 51.5547, 0) along direction (0, 0, -1) blind 1.8 on bodies 5 bodies 5
extrude "Extrusion49" cut 1 faces at (24.6941, 10.0913, 0) along direction (0, 0, -1) blind 1.8 on bodies 5 bodies 5
extrude "Extrusion50" cut 1 faces at (-3.5292, 34.4453, 0) along direction (0, 0, -1) blind 1.8 on bodies 5 bodies 5
sketch "Skizze28" plane through (0, 0, -1.8) normal (0, 0, 1) x (-1, 0, 0)
  circle A0 centre (-45.8, -5.1408) radius 2.5
  circle A1 centre (-4.2, -5.1408) radius 2.5
  arc A2 (15.25, 1.0661) -> (10.25, 6.0661) centre (10.25, 1.0661) ccw
  line L0 (10.25, 6.0661) -> (-60.25, 6.0661)
  arc A3 (-60.25, 6.0661) -> (-65.25, 1.0661) centre (-60.25, 1.0661) ccw
  line L1 (-65.25, 1.0661) -> (-65.25, -87.0661)
  arc A4 (-65.25, -87.0661) -> (-60.25, -92.0661) centre (-60.25, -87.0661) ccw
  line L2 (-60.25, -92.0661) -> (10.25, -92.0661)
  arc A5 (10.25, -92.0661) -> (15.25, -87.0661) centre (10.25, -87.0661) ccw
  line L3 (15.25, -87.0661) -> (15.25, 1.0661)
  line L4 (3.5, -17.2422) -> (3.5, -68.7965)
  ellipse E0 centre (5.45, -73.45) end of major axis (10.1633, -68.9215) minor radius 4.9 (2, -69.97) -> (2, -78.8418) ccw
  line L5 (3.5, -79.1841) -> (3.5, -84)
  arc A6 (-2, -89.5) -> (3.5, -84) centre (-2, -84) ccw
  line L6 (-2, -89.5) -> (-48, -89.5)
  arc A7 (-53.5, -84) -> (-48, -89.5) centre (-48, -84) ccw
  line L7 (-53.5, -84) -> (-53.5, -79.2473)
  ellipse E1 centre (-55.45, -73.45) end of major axis (-50.9215, -78.1633) minor radius 4.9 (-52, -78.8857) -> (-52, -69.9695) ccw
  line L8 (-53.5, -68.7578) -> (-53.5, -17.2035)
  ellipse E2 centre (-55.45, -12.55) end of major axis (-60.1633, -17.0785) minor radius 4.9 (-53.5, -6.8159) -> (-53.5, -17.2035) ccw
  line L9 (-53.5, -6.8159) -> (-53.5, -2)
  arc A8 (-48, 3.5) -> (-53.5, -2) centre (-48, -2) ccw
  line L10 (-48, 3.5) -> (-43, 3.5)
  line L11 (-43, 3.5) -> (-43, 2)
  line L12 (-43, 2) -> (-48, 2)
  arc A9 (-48, 2) -> (-52, -2) centre (-48, -2) ccw
  line L13 (-52, -2) -> (-52, -7.1582)
  ellipse E3 centre (-55.45, -12.55) end of major axis (-60.1633, -17.0785) minor radius 4.9 (-52, -16.03) -> (-52, -7.1582) ccw
  line L14 (2, -84) -> (2, -78.8418)
  ellipse E4 centre (5.45, -12.55) end of major axis (0.9215, -7.8367) minor radius 4.9 (2, -7.1143) -> (2, -16.0305) ccw
  line L15 (2, -7.1143) -> (2, -2)
  arc A10 (2, -2) -> (-2, 2) centre (-2, -2) ccw
  line L16 (-2, 2) -> (-7, 2)
  line L17 (-7, 2) -> (-7, 3.5)
  line L18 (-7, 3.5) -> (-2, 3.5)
  arc A11 (3.5, -2) -> (-2, 3.5) centre (-2, -2) ccw
  line L19 (3.5, -2) -> (3.5, -6.7527)
  ellipse E5 centre (5.45, -12.55) end of major axis (0.9215, -7.8367) minor radius 4.9 (3.5, -17.2422) -> (3.5, -6.7527) ccw
  circle A12 centre (-25, -43) radius 15
  circle A13 centre (-25, -43) radius 26.75
  circle A14 centre (-4.2, -82.6408) radius 2.5
  circle A15 centre (-45.8, -82.6408) radius 2.5
  circle A16 centre (-25, -43) radius 26.75
  line L20 (-52, -16.03) -> (-52, -69.9695)
  line L21 (-52, -78.8857) -> (-52, -84)
  arc A17 (-52, -84) -> (-48, -88) centre (-48, -84) ccw
  line L22 (-48, -88) -> (-2, -88)
  arc A18 (-2, -88) -> (2, -84) centre (-2, -84) ccw
  line L23 (2, -69.97) -> (2, -16.0305)
  ellipse E6 centre (5.45, -73.45) end of major axis (10.1633, -68.9215) minor radius 4.9 (3.5, -79.1841) -> (3.5, -68.7965) ccw
  ellipse E7 centre (-55.45, -73.45) end of major axis (-50.9215, -78.1633) minor radius 4.9 (-53.5, -68.7578) -> (-53.5, -79.2473) ccw
extrude "Extrusion51" add sketch "Skizze28" against normal blind 2 contours A14 bodies 5
sketch "Skizze29" plane through (0, 0, -1.8) normal (0, 0, -1) x (1, 0, 0)
  arc A0 (-10.25, 6.0661) -> (-15.25, 1.0661) centre (-10.25, 1.0661) ccw
  line L0 (-15.25, 1.0661) -> (-15.25, -87.0661)
  arc A1 (-15.25, -87.0661) -> (-10.25, -92.0661) centre (-10.25, -87.0661) ccw
  line L1 (-10.25, -92.0661) -> (60.25, -92.0661)
  arc A2 (60.25, -92.0661) -> (65.25, -87.0661) centre (60.25, -87.0661) ccw
  line L2 (65.25, -87.0661) -> (65.25, 1.0661)
  arc A3 (65.25, 1.0661) -> (60.25, 6.0661) centre (60.25, 1.0661) ccw
  line L3 (60.25, 6.0661) -> (-10.25, 6.0661)
  line L4 (-3.55, -84) -> (-3.55, -2)
  arc A4 (2, 3.55) -> (-3.55, -2) centre (2, -2) ccw
  line L5 (2, 3.55) -> (48, 3.55)
  arc A5 (53.55, -2) -> (48, 3.55) centre (48, -2) ccw
  line L6 (53.55, -2) -> (53.55, -84)
  arc A6 (48, -89.55) -> (53.55, -84) centre (48, -84) ccw
  line L7 (48, -89.55) -> (2, -89.55)
  arc A7 (-3.55, -84) -> (2, -89.55) centre (2, -84) ccw
  line L8 (-10.25, -92.0661) -> (60.25, -92.0661)
  arc A8 (-15.25, -87.0661) -> (-10.25, -92.0661) centre (-10.25, -87.0661) ccw
  line L9 (-15.25, 1.0661) -> (-15.25, -87.0661)
  arc A9 (-10.25, 6.0661) -> (-15.25, 1.0661) centre (-10.25, 1.0661) ccw
  line L10 (60.25, 6.0661) -> (-10.25, 6.0661)
  arc A10 (65.25, 1.0661) -> (60.25, 6.0661) centre (60.25, 1.0661) ccw
  line L11 (65.25, -87.0661) -> (65.25, 1.0661)
  arc A11 (60.25, -92.0661) -> (65.25, -87.0661) centre (60.25, -87.0661) ccw
  line L12 (63.75, -87.0661) -> (63.75, 1.0661)
  arc A12 (63.75, 1.0661) -> (60.25, 4.5661) centre (60.25, 1.0661) ccw
  line L13 (60.25, 4.5661) -> (-10.25, 4.5661)
  arc A13 (-10.25, 4.5661) -> (-13.75, 1.0661) centre (-10.25, 1.0661) ccw
  line L14 (-13.75, 1.0661) -> (-13.75, -87.0661)
  arc A14 (-13.75, -87.0661) -> (-10.25, -90.5661) centre (-10.25, -87.0661) ccw
  line L15 (-10.25, -90.5661) -> (60.25, -90.5661)
  arc A15 (60.25, -90.5661) -> (63.75, -87.0661) centre (60.25, -87.0661) ccw
  arc A16 (60.25, -90.4161) -> (63.6, -87.0661) centre (60.25, -87.0661) ccw
  line L16 (63.6, -87.0661) -> (63.6, 1.0661)
  arc A17 (63.6, 1.0661) -> (60.25, 4.4161) centre (60.25, 1.0661) ccw
  line L17 (60.25, 4.4161) -> (-10.25, 4.4161)
  arc A18 (-10.25, 4.4161) -> (-13.6, 1.0661) centre (-10.25, 1.0661) ccw
  line L18 (-13.6, 1.0661) -> (-13.6, -87.0661)
  arc A19 (-13.6, -87.0661) -> (-10.25, -90.4161) centre (-10.25, -87.0661) ccw
  line L19 (-10.25, -90.4161) -> (60.25, -90.4161)
  dimension "d227" = -1.5
  dimension "d228" = -1.65
extrude "Extrusion52" cut sketch "Skizze29" along normal blind 7 contours A0 L0 A1 L1 A2 L2 A3 L3 L8 A8 L9 A9 L10 A10 L11 A11 | L12 A12 L13 A13 L14 A14 L15 A15 bodies 5
extrude "Extrusion4''" add sketch "Skizze29" along normal blind 3.7 contours A0 L0 A1 L1 A2 L2 A3 L3 L8 A8 L9 A9 L10 A10 L11 A11 bodies 4 in component "Outer Body"
extrude "Extrusion5" cut 1 faces at (60.35, 56.6667, -1.8) along direction (0, 0, 1) blind 0.1 on bodies 4 bodies 4 in component "Outer Body"
extrude "Extrusion6'" cut 1 faces at (54.7167, 29.3333, 10.6) along direction (0, 0, -1) blind 0.12 on bodies 4 bodies 4 in component "Outer Body"
extrude "Extrusion7'" add 1 faces at (54.0167, 29.3333, 10.4) along direction (0, 0, 1) blind 0.1 on bodies 4 bodies 4 in component "Outer Body"
extrude "Extrusion8'" cut 1 faces at (-11.85, 56.6667, 10.5) along direction (0, 0, -1) blind 4 on bodies 4 bodies 4 in component "Outer Body"
move_face "Flächen versetzen5" offset 3.5 1 faces at (51.6171, 45.6634, -22.9333) on bodies 5
move_face "Flächen versetzen6" offset -3.5 1 faces at (53.7143, 41.5669, -25.5) on bodies 5
move_face "Flächen versetzen7" offset -8 1 faces at (39.9255, 44.4935, -34.8333) on bodies 5
extrude "Extrusion53" cut 1 faces at (49.406, 41.7456, -35.5) along direction (0, 0, 1) blind 15 on bodies 5 bodies 5
extrude "Extrusion9'" add 1 faces at (17.3333, 77.4, 10.1667) along direction (0, -1, 0) blind 1.3 on bodies 4 bodies 4 in component "Outer Body"
extrude "Extrusion10'" add 1 faces at (48, 56.6333, 9.8333) along direction (-1, 0, 0) blind 0.8 on bodies 4 bodies 4 in component "Outer Body"
extrude "Extrusion11'" add 1 faces at (2, 37.1667, 9.8333) along direction (1, 0, 0) blind 0.8 on bodies 4 bodies 4 in component "Outer Body"